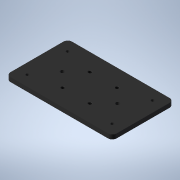
# Autodesk Inventor part: 31000133platte
Saved by Autodesk Inventor 2021 (Build 250183000, 183)
## iProperties
Created: 2025-06-23
Part Number: 31000133platte
Material: Generic
Catalog Web Link: www.cadenas.de
Description: base stand BZB-Accessories
Vendor: RNA
Document SubType Name: Modeling
Designer: psAdmin
Manufacturer: RNA
Mass: 357.401 g
Surface Area: 814.357 cm^2
Volume: 357.401 cm^3
Density: 1 g/cm^3
Appearance: PSOLRGB-175-175-175
Category: PARTsolutions
Company: RNA
Title: 31000133platte
Author: Cadenas PARTsolutions
Comments: Accessories
PSOL_IDENT_0: {$CADENAS_DATA/23d-libs/rna/bunker/zubehoer/parts/bzb_plate.prj},177 {VTYP=3D},{NB=31000133platte},{
PSOL_IDENT_1: LINA=31000133platte},{NN=base stand BZB},{DATE=06.06.2017 11:57:03},{GEOMDATE=02.05.2017 08:45:00},{
PSOL_IDENT_2: VERSION=},{LINEID=200},{WBVAR=},{WBNUMERIC=}  {NB=31000133platte},{LINA=31000133platte},{KT=DUMMY},{
PSOL_IDENT_3: CNSORDERNO=31000133},{KOMP=Bodenständer BZB 550-900mm BVL3},{TYP=BVL3},{VERS=1},{B=10},{ROW=1}
NB: 31000133platte
NN: base stand BZB
NT: Accessories
NBSYN: $CNSORDERNO.platte
LINA: 31000133platte
CATALOG: Rhein-Nadel-Automation
CNSORDERNO: 31000133
KOMP: Bodenständer BZB 550-900mm BVL3
TYP: BVL3
VERS: 1
B: 10
ROW: 1
SUPPLIER: RNA
ARTICLENO: 31000133platte
BOMINFO: 31000133platte
CREATOR: CADENAS GmbH
Autodesk Inventor part; units mm, degrees
sketch "Sketch_1" plane through (0, 0, 0) normal (0, 1, 0) x (-1, 0, 0)
  arc A0 (125, 62.5) -> (115, 72.5) centre (115, 62.5) ccw
  line L0 (115, 72.5) -> (-115, 72.5)
  arc A1 (-115, 72.5) -> (-125, 62.5) centre (-115, 62.5) ccw
  line L1 (-125, 62.5) -> (-125, -62.5)
  arc A2 (-125, -62.5) -> (-115, -72.5) centre (-115, -62.5) ccw
  line L2 (-115, -72.5) -> (115, -72.5)
  arc A3 (115, -72.5) -> (125, -62.5) centre (115, -62.5) ccw
  line L3 (125, -62.5) -> (125, 62.5)
  circle A4 centre (-100, -47.5) radius 3.5
  circle A5 centre (-100, 47.5) radius 3.5
  circle A6 centre (-65, 0) radius 4.5
  circle A7 centre (65, 0) radius 4.5
  circle A8 centre (100, -47.5) radius 3.5
  circle A9 centre (100, 47.5) radius 3.5
  constraints: 10 centre point, 8 end point, 8 point on circle
extrude "Extrusion1" add sketch "Sketch_1" along normal blind 10
sketch "Sketch_9" plane through (0, 0, -32) normal (0, 0, 1) x (1, 0, 0)
  line L0 (-32, 0) -> (-32, 10)
  line L1 (-32, 10) -> (-28, 10)
  line L2 (-28, 10) -> (-28.6765, 9.3235)
  line L3 (-28.6765, 9.3235) -> (-28.6765, 0.6765)
  line L4 (-28.6765, 0.6765) -> (-28, 0)
  line L5 (-28, 0) -> (-32, 0)
  line L6 (-32, 0) -> (-32, 10)
  constraints: 14 end point
revolve "Revolution1" cut sketch "Sketch_9" angle 360 about axis through (-32, 0, -32) along (0, -1, 0)
thread "Thread1" size "M8x1.25" class "6H" standard "ISO Metric profile" full length
sketch "Sketch_10" plane through (0, 0, -32) normal (0, 0, 1) x (1, 0, 0)
  line L0 (32, 0) -> (32, 10)
  line L1 (32, 10) -> (36, 10)
  line L2 (36, 10) -> (35.3235, 9.3235)
  line L3 (35.3235, 9.3235) -> (35.3235, 0.6765)
  line L4 (35.3235, 0.6765) -> (36, 0)
  line L5 (36, 0) -> (32, 0)
  line L6 (32, 0) -> (32, 10)
  constraints: 14 end point
revolve "Revolution2" cut sketch "Sketch_10" angle 360 about axis through (32, 0, -32) along (0, -1, 0)
thread "Thread2" size "M8x1.25" class "6H" standard "ISO Metric profile" full length
sketch "Sketch_11" plane through (0, 0, 32) normal (0, 0, 1) x (1, 0, 0)
  line L0 (-32, 0) -> (-32, 10)
  line L1 (-32, 10) -> (-28, 10)
  line L2 (-28, 10) -> (-28.6765, 9.3235)
  line L3 (-28.6765, 9.3235) -> (-28.6765, 0.6765)
  line L4 (-28.6765, 0.6765) -> (-28, 0)
  line L5 (-28, 0) -> (-32, 0)
  line L6 (-32, 0) -> (-32, 10)
  constraints: 14 end point
revolve "Revolution3" cut sketch "Sketch_11" angle 360 about axis through (-32, 0, 32) along (0, -1, 0)
thread "Thread3" size "M8x1.25" class "6H" standard "ISO Metric profile" full length
sketch "Sketch_12" plane through (0, 0, 32) normal (0, 0, 1) x (1, 0, 0)
  line L0 (32, 0) -> (32, 10)
  line L1 (32, 10) -> (36, 10)
  line L2 (36, 10) -> (35.3235, 9.3235)
  line L3 (35.3235, 9.3235) -> (35.3235, 0.6765)
  line L4 (35.3235, 0.6765) -> (36, 0)
  line L5 (36, 0) -> (32, 0)
  line L6 (32, 0) -> (32, 10)
  constraints: 14 end point
revolve "Revolution4" cut sketch "Sketch_12" angle 360 about axis through (32, 0, 32) along (0, -1, 0)
thread "Thread4" size "M8x1.25" class "6H" standard "ISO Metric profile" full length
ref_plane "PLATTE_XY" through (0, 0, 0) normal (0, 1, 0) x (1, 0, 0)
ref_plane "PLATTE_YZ" through (0, 0, 0) normal (1, 0, 0) x (0, 0, -1)
ref_plane "PLATTE_ZX" through (0, 0, 0) normal (0, 0, -1) x (0, 1, 0)
body "Solid1"
